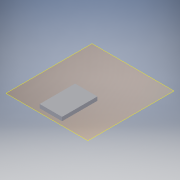
# Autodesk Inventor part: 03_LED
Saved by Autodesk Inventor 2016 (Build 200138000, 138)
## iProperties
Created: 2016-11-08
Part Number: 03_LED
Material: Generisch
Document SubType Name: Modeling
Designer: Bene
Density: 1 g/cm^3
Appearance: Weiß
Author: Bene
Autodesk Inventor part; units mm, degrees
ref_plane "YZ Plane" through (0, 0, 0) normal (1, 0, 0) x (0, 1, 0)
ref_plane "XZ Plane" through (0, 0, 0) normal (0, 1, 0) x (-1, 0, 0)
ref_plane "XY Plane" through (0, 0, 0) normal (0, 0, 1) x (1, 0, 0)
ref_plane "Arbeitsebene1" through (0, 0, 0) normal (0, 0, 1) x (1, 0, 0)
sketch "Skizze1" plane through (0, 0, 0) normal (0, 0, 1) x (1, 0, 0)
  line L0 (0, 0) -> (40, 0) projected
  line L1 (40, 0) -> (40, 42) projected
  line L2 (0, 42) -> (40, 42) projected
  line L3 (0, 0) -> (0, 42) projected
  line L4 (14, 19) -> (26, 19)
  line L5 (26, 19) -> (26, 0)
  line L6 (26, 0) -> (14, 0)
  line L7 (14, 0) -> (14, 19)
  line L8 (14, 19) -> (26, 0) construction
  line L9 (26, 19) -> (14, 0) construction
  point P0 (20, 9.5)
  dimension "d0" = 12
  dimension "d1" = 19
  dimension "d3" = 20
  constraints: 12 end point, 2 midpoint, 2 parallel, 1 horizontal, 1 perpendicular, 1 point on line
  measures "d0" distance of L5.end L6.end
  measures "d1" distance of L4.end L5.end
  measures "d3" distance from line of L3 point (20, 9.5)
extrude "Extrusion1" add sketch "Skizze1" along normal blind 2 contours L7 L4 L5 L0
